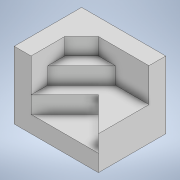
# Autodesk Inventor part: 零件19
Saved by Autodesk Inventor 2020 (Build 240168000, 168)
## iProperties
Created: 2020-12-11
Part Number: 零件19
Material: 一般
Document SubType Name: Modeling
Designer: USER
Density: 1 g/cm^3
Appearance: 預設
Author: USER
Autodesk Inventor part; units mm, degrees
ref_plane "YZ Plane" through (0, 0, 0) normal (1, 0, 0) x (0, 1, 0)
ref_plane "XZ Plane" through (0, 0, 0) normal (0, 1, 0) x (-1, 0, 0)
ref_plane "XY Plane" through (0, 0, 0) normal (0, 0, 1) x (1, 0, 0)
sketch "草圖1" plane through (0, 0, 0) normal (0, 0, 1) x (1, 0, 0)
  line L0 (25, -20) -> (-25, -20)
  line L1 (-25, -20) -> (-25, 20)
  line L2 (-25, 20) -> (25, 20)
  line L3 (25, 20) -> (25, -20)
  line L4 (25, -20) -> (-25, 20) construction
  line L5 (-25, -20) -> (25, 20) construction
  point P0 (0, 0)
  dimension "d0" = 40
  dimension "d1" = 50
  constraints: 12 end point, 2 midpoint, 2 parallel, 1 horizontal, 1 perpendicular
  measures "d0" distance between parallel lines of L0 L2
  measures "d1" distance between parallel lines of L3 L1
extrude "擠出1" add sketch "草圖1" along normal blind 40
sketch "草圖2" plane through (-25, 20, 0) normal (0, 1, 0) x (1, 0, 0)
  line L0 (50, -40) -> (0, -40) projected
  line L1 (50, 0) -> (50, -40) projected
  line L2 (0, 0) -> (0, -40) projected
  line L3 (50, 0) -> (0, 0) projected
  line L4 (0, -40) -> (50, -40) projected
  line L5 (50, -40) -> (30, -20)
  line L6 (30, -20) -> (10, -40)
  line L7 (10, -40) -> (50, -40)
  line L8 (50, 0) -> (0, 0) projected
  line L9 (0, 0) -> (0, -40) projected
  line L10 (50, -40) -> (0, -40) projected
  line L11 (50, 0) -> (50, -40) projected
  point P0 (25, 0)
  dimension "d4" = 10
  dimension "d5" = 20
  dimension "d6" = 20
  constraints: 6 end point, 1 point on line
  measures "d4" distance of L0.end L6.end
  measures "d5" distance from line of L0 L5.end
  measures "d6" distance from line of L1 L5.end
extrude "擠出2" cut sketch "草圖2" against normal blind 30 contours L0 L6 L5
sketch "草圖3" plane through (-25, 20, 0) normal (0, 1, 0) x (1, 0, 0)
  line L0 (0, -40) -> (50, -40) projected
  line L1 (10, -40) -> (10, -30)
  line L2 (10, -30) -> (30, -10)
  line L3 (30, -10) -> (50, -10)
  line L4 (50, 0) -> (50, -40) projected
  line L5 (50, 0) -> (0, 0) projected
  line L6 (0, 0) -> (0, -40) projected
  point P0 (25, 0)
  dimension "d9" = 10
  dimension "d10" = 10
  dimension "d11" = 10
  dimension "d12" = 20
  constraints: 6 end point, 2 point on line, 1 perpendicular, 1 vertical
  measures "d9" distance from line of L0 L1.end
  measures "d10" distance between parallel lines of L3 L5
  measures "d11" distance between parallel lines of L6 L1
  measures "d12" distance from line of L4 L2.end
extrude "擠出3" cut sketch "草圖3" against normal blind 20 contours L1 L2 L3 L4 L0
sketch "草圖4" plane through (-25, 20, 0) normal (0, 1, 0) x (1, 0, 0)
  line L0 (10, -40) -> (10, -30) projected
  line L1 (10, -30) -> (10, -20)
  line L2 (10, -20) -> (20, -10)
  line L3 (30, -10) -> (50, -10) projected
  line L4 (20, -10) -> (30, -10)
  line L5 (30, -10) -> (50, -10) projected
  line L6 (10, -30) -> (30, -10)
  line L7 (10, -30) -> (30, -10) projected
  point P0 (25, 0)
  dimension "d15" = 10
  dimension "d16" = 10
  constraints: 8 end point, 2 point on line, 1 collinear, 1 vertical
  measures "d15" distance of L3.start L2.end
  measures "d16" distance of L0.end L1.end
extrude "擠出4" cut sketch "草圖4" against normal blind 10
